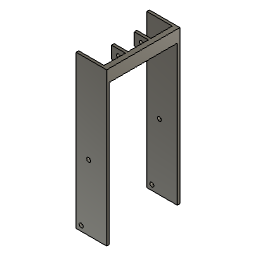
Suspension Plate (2) (Autodesk Fusion 360 design; units mm, degrees)
Autodesk Fusion 360 part; units mm, degrees
sketch "Sketch1" plane through (0, 0, 0) normal (0, 1, 0) x (1, 0, 0)
  line L0 (0, 0) -> (18.5729, 0) construction
  line L1 (18.5729, 0) -> (18.5729, -151.264) construction
  line L2 (18.5729, -151.264) -> (0, -151.264) construction
  line L3 (0, -151.264) -> (0, 0) construction
  line L4 (0, 0) -> (18.5729, -151.264) construction
  line L5 (0, 0) -> (43.3367, -352.9494) construction
  line L6 (-12.7, 12.7) -> (63.5, 12.7)
  line L7 (63.5, 12.7) -> (63.5, -368.3)
  line L8 (63.5, -368.3) -> (-12.7, -368.3)
  line L9 (-12.7, -368.3) -> (-12.7, 12.7)
  circle A0 centre (0, 0) radius 5
  circle A1 centre (18.5729, -151.264) radius 5
  circle A2 centre (43.3367, -352.9494) radius 4.7625
  line L10 (63.5, -368.3) -> (50.8, -368.3)
  line L11 (50.8, -368.3) -> (50.8, -337.82)
  line L12 (50.8, -337.82) -> (63.5, -337.82)
  line L13 (63.5, -337.82) -> (63.5, -368.3)
  line L14 (50.8, -353.06) -> (63.5, -353.06)
  dimension "d7" = 18.5729
  dimension "d8" = 151.264
  dimension "d9" = 355.6
  dimension "d10" = 381
  dimension "d11" = 76.2
  dimension "d13" = 12.7
  dimension "d14" = 12.7
  dimension "d15" = 10
  dimension "d16" = 10
  dimension "d19" = 9.525
  dimension "d22" = 30.48
  dimension "d23" = 12.7
  constraint horizontal L0
  constraint vertical L1
  constraint horizontal L2
  constraint vertical L3
  constraint coincident L0.start L3.end
  constraint parallel L4 L5
  constraint horizontal L6
  constraint vertical L7
  constraint horizontal L8
  constraint vertical L9
  constraint coincident L1.end L2.start
  constraint coincident L5.end A2.centre
  constraint horizontal L10
  constraint vertical L11
  constraint horizontal L12
  constraint vertical L13
  constraint midpoint L11 L14.start
  constraint midpoint L13 L14.end
  measures "d7" distance of L1.end L2.end
  measures "d8" distance of L0.start L2.end
  measures "d9" distance of L0.start L5.end
  measures "d10" distance of L6.end L7.end
  measures "d11" distance of L6.start L6.end
  measures "d13" distance of L3 L9
  measures "d14" distance of L0 L6
  measures "d15" diameter of A0
  measures "d16" diameter of A1
  measures "d19" diameter of A2
  measures "d22" distance of L10.end L11.end
  measures "d23" distance of L11.end L12.end
extrude "Extrude1" add sketch "Sketch1" along normal blind 5.08 contours L6 L7 L8 L9 L11 L12 | L7 L11 L12 L13 L14 | L7 L8 L10 L11 L13 L14 | A2
extrude "Extrude3" add sketch "Sketch1" against normal blind 170.18 contours L7 L11 L12 L13 L14 | L7 L8 L10 L11 L13 L14
sketch "Sketch2" plane through (50.8, 0, 0) normal (-1, 0, 0) x (0, -1, 0)
  line L0 (0, 368.3) -> (0, 337.82)
  line L1 (0, 337.82) -> (170.18, 337.82)
  line L2 (170.18, 337.82) -> (170.18, 368.3)
  line L3 (170.18, 368.3) -> (0, 368.3)
  line L4 (85.09, 337.82) -> (85.09, 368.3)
  line L5 (170.18, 353.06) -> (0, 353.06)
  line L6 (59.69, 348.2975) -> (110.49, 348.2975) construction
  line L7 (110.49, 348.2975) -> (110.49, 357.8225) construction
  line L8 (110.49, 357.8225) -> (59.69, 357.8225) construction
  line L9 (59.69, 357.8225) -> (59.69, 348.2975) construction
  line L10 (59.69, 353.06) -> (110.49, 353.06)
  line L11 (85.09, 357.8225) -> (85.09, 348.2975)
  line L12 (110.49, 368.3) -> (115.57, 368.3)
  line L13 (115.57, 368.3) -> (115.57, 337.82)
  line L14 (115.57, 337.82) -> (110.49, 337.82)
  line L15 (110.49, 337.82) -> (110.49, 368.3)
  line L16 (54.61, 368.3) -> (54.61, 337.82)
  line L17 (59.69, 337.82) -> (59.69, 368.3)
  line L18 (59.69, 368.3) -> (54.61, 368.3)
  line L19 (54.61, 337.82) -> (59.69, 337.82)
  dimension "d26" = 9.525
  dimension "d27" = 50.8
  dimension "d28" = 30.48
  dimension "d29" = 85.09
  dimension "d30" = 5.08
  dimension "d31" = 5.08
  dimension "d32" = 30.48
  constraint midpoint L1 L4.start
  constraint midpoint L3 L4.end
  constraint midpoint L2 L5.start
  constraint midpoint L0 L5.end
  constraint horizontal L6
  constraint vertical L7
  constraint horizontal L8
  constraint vertical L9
  constraint midpoint L9 L10.start
  constraint midpoint L7 L10.end
  constraint midpoint L8 L11.start
  constraint midpoint L6 L11.end
  constraint horizontal L12
  constraint vertical L13
  constraint horizontal L14
  constraint vertical L15
  constraint coincident L3 L12.start
  constraint symmetric L4 L12.start L17.end
  constraint symmetric L4 L12.end L16.start
  constraint symmetric L4 L13.end L16.end
  constraint symmetric L4 L14.end L17.start
  measures "d26" distance of L6.start L8.end
  measures "d27" distance of L6.start L6.end
  measures "d29" distance of L2 L11
  measures "d30" distance of L12.start L12.end
  measures "d31" distance of L7 L13
  measures "d32" distance of L12.end L13.end
extrude "Extrude4" add sketch "Sketch2" along normal blind 34.925 contours L3 L5 L16 L17 L18 | L1 L5 L16 L17 L19 | L3 L5 L12 L13 L15 | L1 L5 L13 L14 L15
hole "Hole1" at (33.3375, -59.69, 353.06) direction (0, 1, 0) diameter 9.525 depth 10.16 tip angle 118
hole "Hole2" at (33.3375, -115.57, 353.06) direction (0, 1, 0) diameter 9.525 depth 10.16 tip angle 118
sketch "Sketch3" plane through (0, -170.18, 0) normal (0, -1, 0) x (1, 0, 0)
  line L0 (50.8, 337.82) -> (63.5, 337.82)
  line L1 (63.5, 337.82) -> (63.5, 368.3)
  line L2 (63.5, 368.3) -> (50.8, 368.3)
  line L3 (50.8, 368.3) -> (50.8, 337.82)
  line L4 (63.5, 368.3) -> (-12.7, 368.3)
  line L5 (-12.7, 368.3) -> (-12.7, -12.7)
  line L6 (-12.7, -12.7) -> (63.5, -12.7)
  line L7 (63.5, -12.7) -> (63.5, 368.3)
  line L8 (0, 0) -> (18.5674, 0) construction
  line L9 (18.5674, 0) -> (18.5674, 151.257) construction
  line L10 (18.5674, 151.257) -> (0, 151.257) construction
  line L11 (0, 151.257) -> (0, 0) construction
  circle A0 centre (0, 0) radius 5
  line L12 (0, 0) -> (18.5674, 151.257) construction
  line L13 (0, 0) -> (43.3261, 352.9507) construction
  circle A1 centre (43.3261, 352.9507) radius 4.7625
  circle A2 centre (18.5674, 151.257) radius 5
  dimension "d41" = 381
  dimension "d42" = 76.2
  dimension "d43" = 151.257
  dimension "d44" = 18.5674
  dimension "d45" = 10
  dimension "d46" = 355.6
  dimension "d47" = 9.525
  dimension "d48" = 10
  constraint horizontal L4
  constraint vertical L5
  constraint horizontal L6
  constraint vertical L7
  constraint coincident L1.end L2.start
  constraint horizontal L8
  constraint vertical L9
  constraint horizontal L10
  constraint vertical L11
  constraint coincident L8.start L11.end
  constraint parallel L12 L13
  constraint coincident L13.end A1.centre
  constraint coincident L9.end L10.start
  measures "d41" distance of L1.end L6.end
  measures "d42" distance of L1.end L4.end
  measures "d43" distance of L8.start L10.end
  measures "d44" distance of L8.start L8.end
  measures "d45" diameter of A0
  measures "d46" distance of L8.start L13.end
  measures "d47" diameter of A1
  measures "d48" diameter of A2
extrude "Extrude5" add 1 faces at (23.1881, 5.08, 297.6201) along direction (0, 1, 0) blind 1.27
extrude "Extrude6" add 1 faces at (20.1128, -54.61, 353.1786) along direction (0, 1, 0) blind 1.27
extrude "Extrude7" add 1 faces at (20.1128, -115.57, 353.1786) along direction (0, -1, 0) blind 1.27
extrude "Extrude8" add sketch "Sketch3" along normal blind 6.35 contours L0 L1 L2 L3 L4 L7 | L0 L3 L4 L5 L6 L7 | A1
equation "d19 = ( 3 / 8 ) * 1 in"
equation "d26 = ( 3 / 8 ) * 1 in"
